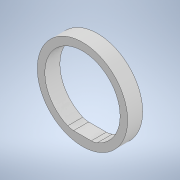
# Autodesk Inventor part: camCircle
Saved by Autodesk Inventor 2021.1 (Build 251245000, 245)
## iProperties
Created: 2020-09-02
Part Number: camCircle
Material: Generic
Document SubType Name: Modeling
Designer: robst
Density: 1 g/cm^3
Appearance: Default
Author: robst
Autodesk Inventor part; units mm, degrees
ref_plane "YZ Plane" through (0, 0, 0) normal (1, 0, 0) x (0, 1, 0)
ref_plane "XZ Plane" through (0, 0, 0) normal (0, 1, 0) x (-1, 0, 0)
ref_plane "XY Plane" through (0, 0, 0) normal (0, 0, 1) x (1, 0, 0)
sketch "Sketch1" plane through (0, 0, 0) normal (0, 0, 1) x (1, 0, 0)
  circle A0 centre (0, 0) radius 15.875
  circle A1 centre (0, 0) radius 19.05
  dimension "d0" = 31.75
  dimension "d1" = 3.175
  constraints: 2 centre point, 2 coincident
  measures "d0" diameter of A0
  measures "d1" radial gap between concentric circles of A1 A0
extrude "Extrusion1" add sketch "Sketch1" along normal blind 6.35
sketch "Sketch2" plane through (0, 0, 0) normal (0, 0, -1) x (-1, 0, 0)
  line L0 (0, 0) -> (0, -19.05) construction
  circle A0 centre (0, 0) radius 19.05 construction
  circle A1 centre (0, 0) radius 15.875 construction
  line L1 (0, -15.113) -> (4.8593, -15.113)
  line L2 (0, -15.113) -> (-4.8593, -15.113)
  arc A2 (-4.8593, -15.113) -> (4.8593, -15.113) centre (0, 0) ccw
  dimension "d4" = 0.762
  constraints: 6 end point, 2 point on circle, 1 centre point, 1 coincident, 1 horizontal, 1 point on line, 1 symmetric about line, 1 vertical, 1 vertical alignment, 4 other
extrude "Extrusion2" add sketch "Sketch2" against normal blind 6.35
fillet "Fillet1" radius 6.35 2 edges at (-4.8593, -15.113, 3.175) (4.8593, -15.113, 3.175)
equation "\"d0\" = insideDiameter"
equation "\"d1\" = ringWidth"
equation "\"d2\" = thickness"
equation "\"d5\" = thickness"
equation "\"insideDiameter\" = 31.75"
equation "\"ringWidth\" = 3.175"
equation "\"thickness\" = 6.35"
body "Solid1"
